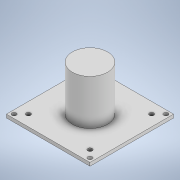
# Autodesk Inventor part: camera_v1
Saved by Autodesk Inventor 2022 (Build 260153000, 153)
## iProperties
Created: 2022-06-05
Part Number: camera_v1
Material: Generic
Document SubType Name: Modeling
Designer: kylem
Density: 1 g/cm^3
Appearance: Default
Author: kylem
Autodesk Inventor part; units mm, degrees
ref_plane "YZ Plane" through (0, 0, 0) normal (1, 0, 0) x (0, 1, 0)
ref_plane "XZ Plane" through (0, 0, 0) normal (0, 1, 0) x (-1, 0, 0)
ref_plane "XY Plane" through (0, 0, 0) normal (0, 0, 1) x (1, 0, 0)
sketch "Sketch1" plane through (0, 0, 0) normal (0, 1, 0) x (-1, 0, 0)
  line L0 (0, 0) -> (38, 0)
  line L1 (38, 0) -> (38, -38)
  line L2 (38, -38) -> (0, -38)
  line L3 (0, -38) -> (0, 0)
  line L4 (19, 0) -> (19, -38)
  line L5 (38, -19) -> (0, -19)
  circle A0 centre (19, -19) radius 8
  line L6 (0, -19) -> (0, -5)
  line L7 (38, -19) -> (38, -5)
  line L8 (38, -19) -> (38, -33)
  line L9 (0, -19) -> (0, -33)
  line L10 (0, -33) -> (38, -33)
  line L11 (38, -5) -> (0, -5)
  line L12 (19, -5) -> (5, -5)
  line L13 (19, -33) -> (33, -33)
  line L14 (33, -33) -> (33, -5)
  line L15 (5, -5) -> (5, -33)
  circle A1 centre (5, -5) radius 1
  circle A2 centre (5, -33) radius 1
  circle A3 centre (33, -33) radius 1
  circle A4 centre (33, -5) radius 1
  dimension "d0" = 38
  dimension "d1" = 38
  dimension "d2" = 16
  dimension "d3" = 14
  dimension "d4" = 14
  dimension "d5" = 14
  dimension "d6" = 14
  dimension "d7" = 14
  dimension "d8" = 14
  dimension "d9" = 28
  dimension "d10" = 28
  dimension "d11" = 2
  dimension "d12" = 2
  dimension "d13" = 2
  dimension "d14" = 2
  constraints: 32 end point, 8 point on line, 7 midpoint, 5 centre point, 4 coincident, 2 parallel, 1 horizontal, 1 perpendicular
  measures "d0" distance of L1.end L2.end
  measures "d1" distance of L0.end L1.end
  measures "d2" diameter of A0
  measures "d3" distance of L5.end L6.end
  measures "d4" distance of L5.start L7.end
  measures "d5" distance of L5.start L8.end
  measures "d6" distance of L5.end L9.end
  measures "d7" distance of L12.start L12.end
  measures "d8" distance of L13.start L13.end
  measures "d9" distance of L13.end L14.end
  measures "d10" distance of L12.end L15.end
  measures "d11" diameter of A1
  measures "d12" diameter of A2
  measures "d13" diameter of A3
  measures "d14" diameter of A4
extrude "Extrusion1" add sketch "Sketch1" along normal blind 1.5 contours L0 L4 L11 A1 L3 | L0 L1 L11 A4 L4 | L11 A1 L15 L5 L3 | L11 A4 L14 L5 A0 L4 | L4 A0 L5 L15 A1 L11 | L5 L15 A2 L10 L3 | L1 L5 L14 A4 L11 | L10 A2 L4 L2 L3 | L5 A0 L4 L10 A2 L15 | L1 L10 A3 L14 L5 | L5 L14 A3 L10 L4 A0 | L1 L2 L4 L10 A3
sketch "Sketch2" plane through (0, 0, 0) normal (0, -1, 0) x (1, 0, 0)
  circle A0 centre (-19, -19) radius 8 projected
  circle A1 centre (-19, -19) radius 8
  point P0 (0, 0)
  constraints: 1 centre point, 1 coincident
extrude "Extrusion2" add sketch "Sketch2" against normal blind 22
sketch "Sketch4" plane through (0, 0, 0) normal (0, -1, 0) x (1, 0, 0)
  line L0 (0, 0) -> (0, -38) projected
  line L1 (0, -19) -> (-38, -19)
  line L2 (-38, -38) -> (-38, 0) projected
  line L3 (0, -38) -> (-38, -38) projected
  line L4 (-19, -38) -> (-19, 0)
  line L5 (-19, -19) -> (-19, -1.75)
  line L6 (-19, -1.75) -> (-1.75, -1.75)
  line L7 (-19, -19) -> (-36.25, -19)
  line L8 (-36.25, -19) -> (-36.25, -36.25)
  circle A0 centre (-1.75, -1.75) radius 1
  circle A1 centre (-36.25, -36.25) radius 1
  circle A2 centre (-1.75, -36.25) radius 1
  circle A3 centre (-36.25, -1.75) radius 1
  dimension "d24" = 17.25
  dimension "d25" = 17.25
  dimension "d26" = 17.25
  dimension "d27" = 17.25
  dimension "d28" = 2
  dimension "d29" = 2
  constraints: 12 end point, 4 centre point, 4 midpoint, 2 coincident, 2 point on line, 2 symmetric about line, 1 parallel, 1 perpendicular, 1 vertical, 2 other
  measures "d24" distance of L5.start L5.end
  measures "d25" distance of L5.end L6.end
  measures "d26" distance of L5.start L7.end
  measures "d27" distance of L7.end L8.end
  measures "d28" diameter of A0
  measures "d29" diameter of A1
extrude "Extrusion4" cut sketch "Sketch4" against normal blind 10 contours A0 | A1 | A2 | A3
body "Solid1"
